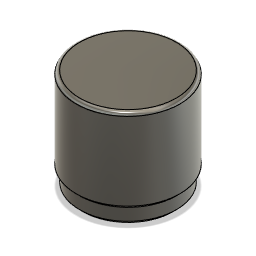
Virgoo Turbocharger Knob v2 (Autodesk Fusion 360 design; units mm, degrees)
Autodesk Fusion 360 part; units mm, degrees
sketch "Sketch1" plane through (0, 0, 0) normal (0, 0, 1) x (1, 0, 0)
  line L0 (0, 3) -> (10, 3)
  line L1 (10, 3) -> (10, 0)
  line L2 (10, 0) -> (14, 0)
  line L3 (14, 0) -> (14, 4.5)
  line L4 (14, 4.5) -> (15, 4.5)
  line L5 (15, 4.5) -> (15, 29)
  line L6 (15, 29) -> (0, 29)
  line L7 (0, 29) -> (0, 3)
  dimension "d1" = 30
  dimension "d2" = 29
  dimension "d3" = 28
  dimension "d4" = 20
  dimension "d5" = 3
  dimension "d6" = 4.5
  constraint horizontal L0
  constraint perpendicular L0 L1
  constraint perpendicular L1 L2
  constraint perpendicular L0 L3
  constraint perpendicular L3 L4
  constraint perpendicular L0 L5
  constraint perpendicular L5 L6
  constraint perpendicular L0 L7
  constraint coincident origin L2
  constraint coincident origin L7
  measures "d2" distance of L2 L6
  measures "d5" distance of L0.end L1.end
  measures "d6" distance of L2.end L3.end
revolve "Revolve1" add sketch "Sketch1" angle 360 about axis through (0, 29, 0) along (0, -1, 0)
chamfer "Chamfer1" distance 1 angle 45 2 edges at (-13.9849, 4.5, -5.4242) (-13.0526, 0, -5.0626)
sketch "Sketch2" plane through (0, 3, 0) normal (0, -1, 0) x (1, 0, 0)
  circle A0 centre (0, 0) radius 10
hole "Hole1" at (0, 3, 0) direction (0, 1, 0) diameter 6 depth 14 tip angle 118
sketch "Sketch3" plane through (0, 0, 0) normal (0, 0, 1) x (1, 0, 0)
  line L0 (13, 0) -> (-13, 0)
  point P0 (0, 9.3)
  dimension "d12" = 9.3
  constraint vertical origin P0
  measures "d12" distance of P0 L0
hole "Hole2" at (0, 9.3, 0) direction (0, 0, -1) diameter 2.529 end through all
thread "Thread1" "ISO Metric profile 3.0 M3x0.5 6H"
chamfer "Chamfer2" distance 0.3 angle 45 1 edges at (1.0848, 3, 2.797)
fillet "Fillet1" radius 1 1 edges at (-13.9849, 29, -5.4242)
